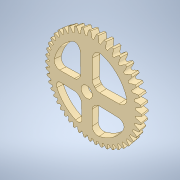
# Autodesk Inventor part: Шестерня катушки
Saved by Autodesk Inventor 2021.1 (Build 251245010, 245A)
## iProperties
Created: 2026-04-13
Part Number: Шестерня катушки
Material: Generic
Document SubType Name: Modeling
Designer: Андрей Тарасов
Density: 1 g/cm^3
Appearance: Default
Author: Андрей Тарасов
Autodesk Inventor part; units mm, degrees
(part 1 of 2)
ref_plane "YZ Plane" through (0, 0, 0) normal (1, 0, 0) x (0, 1, 0)
ref_plane "XZ Plane" through (0, 0, 0) normal (0, 1, 0) x (-1, 0, 0)
ref_plane "XY Plane" through (0, 0, 0) normal (0, 0, 1) x (1, 0, 0)
sketch "Sketch1" plane through (0, 0, 0) normal (0, 0, 1) x (1, 0, 0)
  spline S0 degree 3 poles (-2.1885, 41.8473) (-2.0953, 41.6739) (-1.9088, 41.3271) (-1.6524, 40.7949) (-1.4149, 40.2541) (-1.2364, 39.7953) (-1.1064, 39.4236) (-1.0168, 39.1423) (-0.9329, 38.8591) (-0.8777, 38.6192) (-0.8222, 38.4302) (-0.7732, 38.3167) (-0.7217, 38.2328) (-0.6774, 38.1737) (-0.6275, 38.1192) (-0.5712, 38.0711) (-0.5077, 38.0329) (-0.4402, 38.0029) (-0.3691, 37.9819) (-0.2214, 37.9693) (0, 37.9813) (0.2214, 37.9693) (0.3691, 37.9819) (0.4402, 38.0029) (0.5077, 38.0329) (0.5712, 38.0711) (0.6275, 38.1192) (0.6774, 38.1737) (0.7217, 38.2328) (0.7732, 38.3167) (0.8222, 38.4302) (0.8777, 38.6192) (0.9329, 38.8591) (1.0168, 39.1423) (1.1064, 39.4236) (1.2364, 39.7953) (1.4149, 40.2541) (1.6524, 40.7949) (1.9088, 41.3271) (2.0953, 41.6739) (2.1885, 41.8473) knots 0 0 0 0 0.059055 0.118109 0.177163 0.236216 0.265745 0.295273 0.3248 0.354329 0.36909 0.383846 0.391225 0.398597 0.405969 0.413352 0.420732 0.428104 0.435485 0.442861 0.472389 0.501917 0.509293 0.516674 0.524045 0.531426 0.538808 0.54618 0.553552 0.560931 0.575687 0.590449 0.619977 0.649505 0.679033 0.708561 0.767614 0.826668 0.885723 0.944777 0.944777 0.944777 0.944777
  circle A0 centre (0, 0) radius 37.976 construction
  circle A1 centre (0, 0) radius 37.7362 construction
  circle A2 centre (0, 0) radius 40.158 construction
  circle A3 centre (0, 0) radius 41.9045
  spline S1 degree 3 poles (-7.8664, 41.1595) (-7.7504, 41.0004) (-7.5184, 40.6823) (-7.1919, 40.19) (-6.883, 39.6865) (-6.6436, 39.2563) (-6.4643, 38.9058) (-6.3372, 38.6393) (-6.2155, 38.3701) (-6.1281, 38.14) (-6.0474, 37.9603) (-5.9835, 37.8546) (-5.921, 37.7784) (-5.8691, 37.7259) (-5.8123, 37.6787) (-5.7499, 37.6387) (-5.6818, 37.6096) (-5.6108, 37.589) (-5.5375, 37.5778) (-5.3895, 37.5855) (-5.1718, 37.6275) (-4.9508, 37.6458) (-4.8062, 37.6783) (-4.7386, 37.7089) (-4.6758, 37.7478) (-4.6181, 37.7943) (-4.5689, 37.8496) (-4.5269, 37.9104) (-4.4911, 37.975) (-4.4514, 38.0651) (-4.4184, 38.1842) (-4.3891, 38.379) (-4.3671, 38.6242) (-4.3225, 38.9162) (-4.272, 39.2071) (-4.194, 39.593) (-4.0796, 40.0719) (-3.9179, 40.64) (-3.7363, 41.2021) (-3.5988, 41.5711) (-3.5301, 41.7555) knots 0 0 0 0 0.059055 0.118109 0.177163 0.236216 0.265745 0.295273 0.3248 0.354329 0.36909 0.383846 0.391225 0.398597 0.405969 0.413352 0.420732 0.428104 0.435485 0.442861 0.472389 0.501917 0.509293 0.516674 0.524045 0.531426 0.538808 0.54618 0.553552 0.560931 0.575687 0.590449 0.619977 0.649505 0.679033 0.708561 0.767614 0.826668 0.885723 0.944777 0.944777 0.944777 0.944777
  spline S2 degree 3 poles (-13.3976, 39.705) (-13.2611, 39.5632) (-12.988, 39.2796) (-12.5975, 38.8363) (-12.2229, 38.3797) (-11.9272, 37.9861) (-11.7018, 37.6632) (-11.5396, 37.4165) (-11.3823, 37.1664) (-11.2645, 36.9503) (-11.16, 36.7833) (-11.0823, 36.6872) (-11.01, 36.6203) (-10.9514, 36.5753) (-10.8887, 36.5363) (-10.8215, 36.5052) (-10.75, 36.4856) (-10.6769, 36.4749) (-10.6027, 36.4738) (-10.4572, 36.5016) (-10.2472, 36.5728) (-10.0308, 36.6211) (-9.892, 36.673) (-9.8292, 36.7124) (-9.7723, 36.7596) (-9.7214, 36.8134) (-9.6802, 36.8749) (-9.6468, 36.9409) (-9.6202, 37.0097) (-9.5932, 37.1045) (-9.5767, 37.227) (-9.5742, 37.4239) (-9.5858, 37.6698) (-9.5814, 37.9651) (-9.571, 38.2602) (-9.5461, 38.6532) (-9.498, 39.1431) (-9.4152, 39.728) (-9.3119, 40.3096) (-9.2259, 40.6938) (-9.1829, 40.8859) knots 0 0 0 0 0.059055 0.118109 0.177163 0.236216 0.265745 0.295273 0.3248 0.354329 0.36909 0.383846 0.391225 0.398597 0.405969 0.413352 0.420732 0.428104 0.435485 0.442861 0.472389 0.501917 0.509293 0.516674 0.524045 0.531426 0.538808 0.54618 0.553552 0.560931 0.575687 0.590449 0.619977 0.649505 0.679033 0.708561 0.767614 0.826668 0.885723 0.944777 0.944777 0.944777 0.944777
  spline S3 degree 3 poles (-18.6793, 37.5109) (-18.5248, 37.389) (-18.2156, 37.1452) (-17.7683, 36.7593) (-17.335, 36.3579) (-16.9885, 36.0082) (-16.7213, 35.719) (-16.527, 35.4967) (-16.3371, 35.2703) (-16.1909, 35.0723) (-16.0647, 34.9211) (-15.9747, 34.8365) (-15.8939, 34.7801) (-15.8298, 34.7434) (-15.7623, 34.7133) (-15.6915, 34.6916) (-15.618, 34.682) (-15.5442, 34.6813) (-15.4705, 34.6904) (-15.3301, 34.7377) (-15.1318, 34.8369) (-14.9239, 34.9141) (-14.7935, 34.9844) (-14.7366, 35.0321) (-14.6867, 35.0865) (-14.6436, 35.1468) (-14.6111, 35.2134) (-14.5871, 35.2832) (-14.5701, 35.3551) (-14.5562, 35.4526) (-14.5566, 35.5762) (-14.5809, 35.7716) (-14.6259, 36.0136) (-14.6617, 36.3069) (-14.6916, 36.6006) (-14.7205, 36.9933) (-14.7395, 37.4852) (-14.7372, 38.0759) (-14.714, 38.6662) (-14.6811, 39.0585) (-14.6647, 39.2547) knots 0 0 0 0 0.059055 0.118109 0.177163 0.236216 0.265745 0.295273 0.3248 0.354329 0.36909 0.383846 0.391225 0.398597 0.405969 0.413352 0.420732 0.428104 0.435485 0.442861 0.472389 0.501917 0.509293 0.516674 0.524045 0.531426 0.538808 0.54618 0.553552 0.560931 0.575687 0.590449 0.619977 0.649505 0.679033 0.708561 0.767614 0.826668 0.885723 0.944777 0.944777 0.944777 0.944777
  spline S4 degree 3 poles (-23.6131, 34.618) (-23.4433, 34.5183) (-23.1038, 34.3189) (-22.6082, 33.9974) (-22.1243, 33.6588) (-21.7334, 33.3595) (-21.4293, 33.1094) (-21.2065, 32.9156) (-20.9876, 32.7173) (-20.8158, 32.541) (-20.6702, 32.4084) (-20.5694, 32.3368) (-20.4818, 32.2919) (-20.4132, 32.2643) (-20.3423, 32.2437) (-20.2692, 32.2319) (-20.1951, 32.2323) (-20.1218, 32.2417) (-20.0501, 32.2607) (-19.9175, 32.3267) (-19.7345, 32.452) (-19.539, 32.5568) (-19.4194, 32.6442) (-19.3696, 32.6991) (-19.3275, 32.7599) (-19.2931, 32.8255) (-19.2699, 32.8958) (-19.2556, 32.9683) (-19.2486, 33.0418) (-19.2481, 33.1403) (-19.2653, 33.2627) (-19.316, 33.453) (-19.3935, 33.6866) (-19.4689, 33.9723) (-19.5385, 34.2592) (-19.6207, 34.6443) (-19.7065, 35.1291) (-19.7846, 35.7145) (-19.842, 36.3025) (-19.8628, 36.6957) (-19.8733, 36.8923) knots 0 0 0 0 0.059055 0.118109 0.177163 0.236216 0.265745 0.295273 0.3248 0.354329 0.36909 0.383846 0.391225 0.398597 0.405969 0.413352 0.420732 0.428104 0.435485 0.442861 0.472389 0.501917 0.509293 0.516674 0.524045 0.531426 0.538808 0.54618 0.553552 0.560931 0.575687 0.590449 0.619977 0.649505 0.679033 0.708561 0.767614 0.826668 0.885723 0.944777 0.944777 0.944777 0.944777
  spline S5 degree 3 poles (-28.107, 31.0803) (-27.9252, 31.0046) (-27.5617, 30.8533) (-27.027, 30.6023) (-26.5014, 30.3327) (-26.0734, 30.0894) (-25.7381, 29.8831) (-25.491, 29.7214) (-25.2471, 29.5547) (-25.0529, 29.4035) (-24.8906, 29.2919) (-24.781, 29.2347) (-24.6881, 29.2022) (-24.6164, 29.1842) (-24.5433, 29.1734) (-24.4693, 29.1717) (-24.396, 29.1822) (-24.3246, 29.2015) (-24.2562, 29.23) (-24.1338, 29.3135) (-23.9695, 29.4625) (-23.7902, 29.593) (-23.6836, 29.6959) (-23.6417, 29.7571) (-23.6083, 29.823) (-23.5831, 29.8926) (-23.5698, 29.9655) (-23.5655, 30.0393) (-23.5685, 30.1131) (-23.5814, 30.2107) (-23.6151, 30.3296) (-23.6913, 30.5112) (-23.7999, 30.7321) (-23.9135, 31.0048) (-24.0215, 31.2796) (-24.1553, 31.6499) (-24.3064, 32.1185) (-24.4634, 32.6879) (-24.6004, 33.2625) (-24.6746, 33.6492) (-24.7117, 33.8426) knots 0 0 0 0 0.059055 0.118109 0.177163 0.236216 0.265745 0.295273 0.3248 0.354329 0.36909 0.383846 0.391225 0.398597 0.405969 0.413352 0.420732 0.428104 0.435485 0.442861 0.472389 0.501917 0.509293 0.516674 0.524045 0.531426 0.538808 0.54618 0.553552 0.560931 0.575687 0.590449 0.619977 0.649505 0.679033 0.708561 0.767614 0.826668 0.885723 0.944777 0.944777 0.944777 0.944777
  spline S6 degree 3 poles (-32.0773, 26.9635) (-31.8869, 26.9133) (-31.5062, 26.8129) (-30.9423, 26.6371) (-30.3849, 26.4415) (-29.9277, 26.2589) (-29.5674, 26.1001) (-29.3006, 25.9736) (-29.0363, 25.8416) (-28.8234, 25.7182) (-28.6474, 25.6298) (-28.531, 25.5881) (-28.4345, 25.5685) (-28.3611, 25.5605) (-28.2872, 25.5597) (-28.2136, 25.5681) (-28.1424, 25.5885) (-28.0744, 25.6173) (-28.0104, 25.6549) (-27.9005, 25.7542) (-27.7581, 25.9243) (-27.5982, 26.0779) (-27.5066, 26.1943) (-27.4734, 26.2607) (-27.4493, 26.3306) (-27.4338, 26.403) (-27.4305, 26.477) (-27.4363, 26.5506) (-27.4493, 26.6233) (-27.4755, 26.7183) (-27.525, 26.8315) (-27.6252, 27.0011) (-27.7629, 27.2052) (-27.9126, 27.4598) (-28.057, 27.7174) (-28.24, 28.066) (-28.4534, 28.5096) (-28.6866, 29.0523) (-28.9005, 29.603) (-29.0266, 29.976) (-29.0897, 30.1625) knots 0 0 0 0 0.059055 0.118109 0.177163 0.236216 0.265745 0.295273 0.3248 0.354329 0.36909 0.383846 0.391225 0.398597 0.405969 0.413352 0.420732 0.428104 0.435485 0.442861 0.472389 0.501917 0.509293 0.516674 0.524045 0.531426 0.538808 0.54618 0.553552 0.560931 0.575687 0.590449 0.619977 0.649505 0.679033 0.708561 0.767614 0.826668 0.885723 0.944777 0.944777 0.944777 0.944777
  spline S7 degree 3 poles (-35.4501, 22.3445) (-35.2546, 22.3207) (-34.8638, 22.2731) (-34.2811, 22.1757) (-33.7024, 22.0578) (-33.2246, 21.9391) (-32.846, 21.8309) (-32.5645, 21.7419) (-32.2847, 21.6472) (-32.0569, 21.5539) (-31.8705, 21.4903) (-31.7495, 21.4648) (-31.6512, 21.4585) (-31.5774, 21.4606) (-31.5041, 21.4699) (-31.4323, 21.4882) (-31.3646, 21.5181) (-31.3011, 21.5559) (-31.2429, 21.6019) (-31.1475, 21.7153) (-31.0296, 21.9031) (-30.8921, 22.0771) (-30.8172, 22.2049) (-30.7934, 22.2752) (-30.779, 22.3476) (-30.7735, 22.4215) (-30.7803, 22.4953) (-30.7961, 22.5674) (-30.8189, 22.6377) (-30.8577, 22.7282) (-30.9222, 22.8336) (-31.0446, 22.988) (-31.2087, 23.1714) (-31.3917, 23.4033) (-31.5699, 23.6388) (-31.7986, 23.9593) (-32.0705, 24.3697) (-32.3753, 24.8756) (-32.6622, 25.392) (-32.838, 25.7443) (-32.9259, 25.9205) knots 0 0 0 0 0.059055 0.118109 0.177163 0.236216 0.265745 0.295273 0.3248 0.354329 0.36909 0.383846 0.391225 0.398597 0.405969 0.413352 0.420732 0.428104 0.435485 0.442861 0.472389 0.501917 0.509293 0.516674 0.524045 0.531426 0.538808 0.54618 0.553552 0.560931 0.575687 0.590449 0.619977 0.649505 0.679033 0.708561 0.767614 0.826668 0.885723 0.944777 0.944777 0.944777 0.944777
  spline S8 degree 3 poles (-38.1625, 17.3093) (-37.9656, 17.3123) (-37.5719, 17.3184) (-36.9814, 17.3012) (-36.392, 17.2633) (-35.9025, 17.2107) (-35.5127, 17.155) (-35.2217, 17.1052) (-34.9316, 17.0494) (-34.6932, 16.9881) (-34.4999, 16.9504) (-34.3766, 16.9416) (-34.2784, 16.9488) (-34.2055, 16.9609) (-34.1342, 16.9801) (-34.0655, 17.008) (-34.0025, 17.0468) (-33.9447, 17.093) (-33.8933, 17.1464) (-33.8143, 17.2717) (-33.723, 17.4739) (-33.6105, 17.665) (-33.5537, 17.8018) (-33.5397, 17.8747) (-33.5353, 17.9484) (-33.5399, 18.0223) (-33.5567, 18.0945) (-33.5822, 18.1639) (-33.6143, 18.2303) (-33.6651, 18.3147) (-33.7434, 18.4104) (-33.8856, 18.5466) (-34.0732, 18.706) (-34.2861, 18.9108) (-34.4946, 19.1198) (-34.7649, 19.4062) (-35.0901, 19.7758) (-35.461, 20.2355) (-35.8156, 20.708) (-36.0377, 21.0331) (-36.1487, 21.1956) knots 0 0 0 0 0.059055 0.118109 0.177163 0.236216 0.265745 0.295273 0.3248 0.354329 0.36909 0.383846 0.391225 0.398597 0.405969 0.413352 0.420732 0.428104 0.435485 0.442861 0.472389 0.501917 0.509293 0.516674 0.524045 0.531426 0.538808 0.54618 0.553552 0.560931 0.575687 0.590449 0.619977 0.649505 0.679033 0.708561 0.767614 0.826668 0.885723 0.944777 0.944777 0.944777 0.944777
  spline S9 degree 3 poles (-40.164, 11.9516) (-39.9694, 11.9814) (-39.5802, 12.041) (-38.9928, 12.1044) (-38.4037, 12.1471) (-37.9116, 12.1617) (-37.5179, 12.1596) (-37.2228, 12.1499) (-36.9278, 12.1341) (-36.6833, 12.1058) (-36.4866, 12.0948) (-36.3633, 12.1029) (-36.267, 12.1234) (-36.1964, 12.1453) (-36.1284, 12.174) (-36.0642, 12.211) (-36.007, 12.2581) (-35.9561, 12.3116) (-35.9124, 12.3716) (-35.8512, 12.5065) (-35.7883, 12.7192) (-35.7029, 12.9238) (-35.6652, 13.0671) (-35.6612, 13.1412) (-35.6669, 13.2149) (-35.6816, 13.2875) (-35.7081, 13.3566) (-35.7427, 13.4219) (-35.7836, 13.4834) (-35.8454, 13.5601) (-35.936, 13.6442) (-36.0954, 13.7598) (-36.303, 13.8921) (-36.5417, 14.0661) (-36.7768, 14.2447) (-37.0836, 14.4916) (-37.4561, 14.8135) (-37.8861, 15.2184) (-38.3017, 15.6382) (-38.566, 15.9301) (-38.6982, 16.076) knots 0 0 0 0 0.059055 0.118109 0.177163 0.236216 0.265745 0.295273 0.3248 0.354329 0.36909 0.383846 0.391225 0.398597 0.405969 0.413352 0.420732 0.428104 0.435485 0.442861 0.472389 0.501917 0.509293 0.516674 0.524045 0.531426 0.538808 0.54618 0.553552 0.560931 0.575687 0.590449 0.619977 0.649505 0.679033 0.708561 0.767614 0.826668 0.885723 0.944777 0.944777 0.944777 0.944777
  spline S10 degree 3 poles (-41.4173, 6.3713) (-41.2286, 6.4273) (-40.8511, 6.5394) (-40.2779, 6.6821) (-39.7, 6.8046) (-39.2145, 6.8861) (-38.8242, 6.9377) (-38.5305, 6.9682) (-38.2361, 6.9928) (-37.99, 6.998) (-37.7937, 7.0139) (-37.6726, 7.0387) (-37.58, 7.0721) (-37.5131, 7.1034) (-37.4496, 7.1412) (-37.391, 7.1865) (-37.3407, 7.2409) (-37.2976, 7.3009) (-37.2625, 7.3663) (-37.2202, 7.5083) (-37.1869, 7.7275) (-37.1301, 7.9419) (-37.1123, 8.089) (-37.1185, 8.1629) (-37.1342, 8.2351) (-37.1586, 8.3051) (-37.1942, 8.37) (-37.2374, 8.4299) (-37.2863, 8.4853) (-37.358, 8.5528) (-37.4592, 8.6238) (-37.6329, 8.7166) (-37.8565, 8.8195) (-38.1167, 8.9593) (-38.374, 9.1043) (-38.7114, 9.3071) (-39.1243, 9.5752) (-39.6055, 9.9178) (-40.0744, 10.2771) (-40.376, 10.5303) (-40.5267, 10.6568) knots 0 0 0 0 0.059055 0.118109 0.177163 0.236216 0.265745 0.295273 0.3248 0.354329 0.36909 0.383846 0.391225 0.398597 0.405969 0.413352 0.420732 0.428104 0.435485 0.442861 0.472389 0.501917 0.509293 0.516674 0.524045 0.531426 0.538808 0.54618 0.553552 0.560931 0.575687 0.590449 0.619977 0.649505 0.679033 0.708561 0.767614 0.826668 0.885723 0.944777 0.944777 0.944777 0.944777
  spline S11 degree 3 poles (-41.8991, 0.6723) (-41.7197, 0.7535) (-41.361, 0.9159) (-40.8126, 1.1354) (-40.2568, 1.3354) (-39.7869, 1.4823) (-39.4072, 1.5865) (-39.1204, 1.6567) (-38.8322, 1.7212) (-38.5891, 1.7598) (-38.3968, 1.8023) (-38.2802, 1.8434) (-38.1929, 1.8891) (-38.1309, 1.9292) (-38.0731, 1.9753) (-38.0213, 2.0282) (-37.9789, 2.0889) (-37.9444, 2.1542) (-37.9185, 2.2238) (-37.8959, 2.3702) (-37.8927, 2.5919) (-37.8657, 2.812) (-37.8681, 2.9602) (-37.8843, 3.0326) (-37.9096, 3.102) (-37.9433, 3.1679) (-37.9875, 3.2274) (-38.0385, 3.2809) (-38.0944, 3.3291) (-38.1746, 3.3863) (-38.2845, 3.4428) (-38.4693, 3.5111) (-38.7048, 3.5825) (-38.9817, 3.6856) (-39.2562, 3.7942) (-39.6182, 3.9492) (-40.0637, 4.1586) (-40.5871, 4.4325) (-41.1005, 4.7246) (-41.4338, 4.9343) (-41.6004, 5.0392) knots 0 0 0 0 0.059055 0.118109 0.177163 0.236216 0.265745 0.295273 0.3248 0.354329 0.36909 0.383846 0.391225 0.398597 0.405969 0.413352 0.420732 0.428104 0.435485 0.442861 0.472389 0.501917 0.509293 0.516674 0.524045 0.531426 0.538808 0.54618 0.553552 0.560931 0.575687 0.590449 0.619977 0.649505 0.679033 0.708561 0.767614 0.826668 0.885723 0.944777 0.944777 0.944777 0.944777
  spline S12 degree 3 poles (-41.6004, -5.0392) (-41.4338, -4.9343) (-41.1005, -4.7246) (-40.5871, -4.4325) (-40.0637, -4.1586) (-39.6182, -3.9492) (-39.2562, -3.7942) (-38.9817, -3.6856) (-38.7048, -3.5825) (-38.4693, -3.5111) (-38.2845, -3.4428) (-38.1746, -3.3863) (-38.0944, -3.3291) (-38.0385, -3.2809) (-37.9875, -3.2274) (-37.9433, -3.1679) (-37.9096, -3.102) (-37.8843, -3.0326) (-37.8681, -2.9602) (-37.8657, -2.812) (-37.8927, -2.5919) (-37.8959, -2.3702) (-37.9185, -2.2238) (-37.9444, -2.1542) (-37.9789, -2.0889) (-38.0213, -2.0282) (-38.0731, -1.9753) (-38.1309, -1.9292) (-38.1929, -1.8891) (-38.2802, -1.8434) (-38.3968, -1.8023) (-38.5891, -1.7598) (-38.8322, -1.7212) (-39.1204, -1.6567) (-39.4072, -1.5865) (-39.7869, -1.4823) (-40.2568, -1.3354) (-40.8126, -1.1354) (-41.361, -0.9159) (-41.7197, -0.7535) (-41.8991, -0.6723) knots 0 0 0 0 0.059055 0.118109 0.177163 0.236216 0.265745 0.295273 0.3248 0.354329 0.36909 0.383846 0.391225 0.398597 0.405969 0.413352 0.420732 0.428104 0.435485 0.442861 0.472389 0.501917 0.509293 0.516674 0.524045 0.531426 0.538808 0.54618 0.553552 0.560931 0.575687 0.590449 0.619977 0.649505 0.679033 0.708561 0.767614 0.826668 0.885723 0.944777 0.944777 0.944777 0.944777
  spline S13 degree 3 poles (-40.5267, -10.6568) (-40.376, -10.5303) (-40.0744, -10.2771) (-39.6055, -9.9178) (-39.1243, -9.5752) (-38.7114, -9.3071) (-38.374, -9.1043) (-38.1167, -8.9593) (-37.8565, -8.8195) (-37.6329, -8.7166) (-37.4592, -8.6238) (-37.358, -8.5528) (-37.2863, -8.4853) (-37.2374, -8.4299) (-37.1942, -8.37) (-37.1586, -8.3051) (-37.1342, -8.2351) (-37.1185, -8.1629) (-37.1123, -8.089) (-37.1301, -7.9419) (-37.1869, -7.7275) (-37.2202, -7.5083) (-37.2625, -7.3663) (-37.2976, -7.3009) (-37.3407, -7.2409) (-37.391, -7.1865) (-37.4496, -7.1412) (-37.5131, -7.1034) (-37.58, -7.0721) (-37.6726, -7.0387) (-37.7937, -7.0139) (-37.99, -6.998) (-38.2361, -6.9928) (-38.5305, -6.9682) (-38.8242, -6.9377) (-39.2145, -6.8861) (-39.7, -6.8046) (-40.2779, -6.6821) (-40.8511, -6.5394) (-41.2286, -6.4273) (-41.4173, -6.3713) knots 0 0 0 0 0.059055 0.118109 0.177163 0.236216 0.265745 0.295273 0.3248 0.354329 0.36909 0.383846 0.391225 0.398597 0.405969 0.413352 0.420732 0.428104 0.435485 0.442861 0.472389 0.501917 0.509293 0.516674 0.524045 0.531426 0.538808 0.54618 0.553552 0.560931 0.575687 0.590449 0.619977 0.649505 0.679033 0.708561 0.767614 0.826668 0.885723 0.944777 0.944777 0.944777 0.944777
  spline S14 degree 3 poles (-38.6982, -16.076) (-38.566, -15.9301) (-38.3017, -15.6382) (-37.8861, -15.2184) (-37.4561, -14.8135) (-37.0836, -14.4916) (-36.7768, -14.2447) (-36.5417, -14.0661) (-36.303, -13.8921) (-36.0954, -13.7598) (-35.936, -13.6442) (-35.8454, -13.5601) (-35.7836, -13.4834) (-35.7427, -13.4219) (-35.7081, -13.3566) (-35.6816, -13.2875) (-35.6669, -13.2149) (-35.6612, -13.1412) (-35.6652, -13.0671) (-35.7029, -12.9238) (-35.7883, -12.7192) (-35.8512, -12.5065) (-35.9124, -12.3716) (-35.9561, -12.3116) (-36.007, -12.2581) (-36.0642, -12.211) (-36.1284, -12.174) (-36.1964, -12.1453) (-36.267, -12.1234) (-36.3633, -12.1029) (-36.4866, -12.0948) (-36.6833, -12.1058) (-36.9278, -12.1341) (-37.2228, -12.1499) (-37.5179, -12.1596) (-37.9116, -12.1617) (-38.4037, -12.1471) (-38.9928, -12.1044) (-39.5802, -12.041) (-39.9694, -11.9814) (-40.164, -11.9516) knots 0 0 0 0 0.059055 0.118109 0.177163 0.236216 0.265745 0.295273 0.3248 0.354329 0.36909 0.383846 0.391225 0.398597 0.405969 0.413352 0.420732 0.428104 0.435485 0.442861 0.472389 0.501917 0.509293 0.516674 0.524045 0.531426 0.538808 0.54618 0.553552 0.560931 0.575687 0.590449 0.619977 0.649505 0.679033 0.708561 0.767614 0.826668 0.885723 0.944777 0.944777 0.944777 0.944777
  spline S15 degree 3 poles (-36.1487, -21.1956) (-36.0377, -21.0331) (-35.8156, -20.708) (-35.461, -20.2355) (-35.0901, -19.7758) (-34.7649, -19.4062) (-34.4946, -19.1198) (-34.2861, -18.9108) (-34.0732, -18.706) (-33.8856, -18.5466) (-33.7434, -18.4104) (-33.6651, -18.3147) (-33.6143, -18.2303) (-33.5822, -18.1639) (-33.5567, -18.0945) (-33.5399, -18.0223) (-33.5353, -17.9484) (-33.5397, -17.8747) (-33.5537, -17.8018) (-33.6105, -17.665) (-33.723, -17.4739) (-33.8143, -17.2717) (-33.8933, -17.1464) (-33.9447, -17.093) (-34.0025, -17.0468) (-34.0655, -17.008) (-34.1342, -16.9801) (-34.2055, -16.9609) (-34.2784, -16.9488) (-34.3766, -16.9416) (-34.4999, -16.9504) (-34.6932, -16.9881) (-34.9316, -17.0494) (-35.2217, -17.1052) (-35.5127, -17.155) (-35.9025, -17.2107) (-36.392, -17.2633) (-36.9814, -17.3012) (-37.5719, -17.3184) (-37.9656, -17.3123) (-38.1625, -17.3093) knots 0 0 0 0 0.059055 0.118109 0.177163 0.236216 0.265745 0.295273 0.3248 0.354329 0.36909 0.383846 0.391225 0.398597 0.405969 0.413352 0.420732 0.428104 0.435485 0.442861 0.472389 0.501917 0.509293 0.516674 0.524045 0.531426 0.538808 0.54618 0.553552 0.560931 0.575687 0.590449 0.619977 0.649505 0.679033 0.708561 0.767614 0.826668 0.885723 0.944777 0.944777 0.944777 0.944777
  spline S16 degree 3 poles (-32.9259, -25.9205) (-32.838, -25.7443) (-32.6622, -25.392) (-32.3753, -24.8756) (-32.0705, -24.3697) (-31.7986, -23.9593) (-31.5699, -23.6388) (-31.3917, -23.4033) (-31.2087, -23.1714) (-31.0446, -22.988) (-30.9222, -22.8336) (-30.8577, -22.7282) (-30.8189, -22.6377) (-30.7961, -22.5674) (-30.7803, -22.4953) (-30.7735, -22.4215) (-30.779, -22.3476) (-30.7934, -22.2752) (-30.8172, -22.2049) (-30.8921, -22.0771) (-31.0296, -21.9031) (-31.1475, -21.7153) (-31.2429, -21.6019) (-31.3011, -21.5559) (-31.3646, -21.5181) (-31.4323, -21.4882) (-31.5041, -21.4699) (-31.5774, -21.4606) (-31.6512, -21.4585) (-31.7495, -21.4648) (-31.8705, -21.4903) (-32.0569, -21.5539) (-32.2847, -21.6472) (-32.5645, -21.7419) (-32.846, -21.8309) (-33.2246, -21.9391) (-33.7024, -22.0578) (-34.2811, -22.1757) (-34.8638, -22.2731) (-35.2546, -22.3207) (-35.4501, -22.3445) knots 0 0 0 0 0.059055 0.118109 0.177163 0.236216 0.265745 0.295273 0.3248 0.354329 0.36909 0.383846 0.391225 0.398597 0.405969 0.413352 0.420732 0.428104 0.435485 0.442861 0.472389 0.501917 0.509293 0.516674 0.524045 0.531426 0.538808 0.54618 0.553552 0.560931 0.575687 0.590449 0.619977 0.649505 0.679033 0.708561 0.767614 0.826668 0.885723 0.944777 0.944777 0.944777 0.944777
  spline S17 degree 3 poles (-29.0897, -30.1625) (-29.0266, -29.976) (-28.9005, -29.603) (-28.6866, -29.0523) (-28.4534, -28.5096) (-28.24, -28.066) (-28.057, -27.7174) (-27.9126, -27.4598) (-27.7629, -27.2052) (-27.6252, -27.0011) (-27.525, -26.8315) (-27.4755, -26.7183) (-27.4493, -26.6233) (-27.4363, -26.5506) (-27.4305, -26.477) (-27.4338, -26.403) (-27.4493, -26.3306) (-27.4734, -26.2607) (-27.5066, -26.1943) (-27.5982, -26.0779) (-27.7581, -25.9243) (-27.9005, -25.7542) (-28.0104, -25.6549) (-28.0744, -25.6173) (-28.1424, -25.5885) (-28.2136, -25.5681) (-28.2872, -25.5597) (-28.3611, -25.5605) (-28.4345, -25.5685) (-28.531, -25.5881) (-28.6474, -25.6298) (-28.8234, -25.7182) (-29.0363, -25.8416) (-29.3006, -25.9736) (-29.5674, -26.1001) (-29.9277, -26.2589) (-30.3849, -26.4415) (-30.9423, -26.6371) (-31.5062, -26.8129) (-31.8869, -26.9133) (-32.0773, -26.9635) knots 0 0 0 0 0.059055 0.118109 0.177163 0.236216 0.265745 0.295273 0.3248 0.354329 0.36909 0.383846 0.391225 0.398597 0.405969 0.413352 0.420732 0.428104 0.435485 0.442861 0.472389 0.501917 0.509293 0.516674 0.524045 0.531426 0.538808 0.54618 0.553552 0.560931 0.575687 0.590449 0.619977 0.649505 0.679033 0.708561 0.767614 0.826668 0.885723 0.944777 0.944777 0.944777 0.944777
  spline S18 degree 3 poles (-24.7117, -33.8426) (-24.6746, -33.6492) (-24.6004, -33.2625) (-24.4634, -32.6879) (-24.3064, -32.1185) (-24.1553, -31.6499) (-24.0215, -31.2796) (-23.9135, -31.0048) (-23.7999, -30.7321) (-23.6913, -30.5112) (-23.6151, -30.3296) (-23.5814, -30.2107) (-23.5685, -30.1131) (-23.5655, -30.0393) (-23.5698, -29.9655) (-23.5831, -29.8926) (-23.6083, -29.823) (-23.6417, -29.7571) (-23.6836, -29.6959) (-23.7902, -29.593) (-23.9695, -29.4625) (-24.1338, -29.3135) (-24.2562, -29.23) (-24.3246, -29.2015) (-24.396, -29.1822) (-24.4693, -29.1717) (-24.5433, -29.1734) (-24.6164, -29.1842) (-24.6881, -29.2022) (-24.781, -29.2347) (-24.8906, -29.2919) (-25.0529, -29.4035) (-25.2471, -29.5547) (-25.491, -29.7214) (-25.7381, -29.8831) (-26.0734, -30.0894) (-26.5014, -30.3327) (-27.027, -30.6023) (-27.5617, -30.8533) (-27.9252, -31.0046) (-28.107, -31.0803) knots 0 0 0 0 0.059055 0.118109 0.177163 0.236216 0.265745 0.295273 0.3248 0.354329 0.36909 0.383846 0.391225 0.398597 0.405969 0.413352 0.420732 0.428104 0.435485 0.442861 0.472389 0.501917 0.509293 0.516674 0.524045 0.531426 0.538808 0.54618 0.553552 0.560931 0.575687 0.590449 0.619977 0.649505 0.679033 0.708561 0.767614 0.826668 0.885723 0.944777 0.944777 0.944777 0.944777
  spline S19 degree 3 poles (-19.8733, -36.8923) (-19.8628, -36.6957) (-19.842, -36.3025) (-19.7846, -35.7145) (-19.7065, -35.1291) (-19.6207, -34.6443) (-19.5385, -34.2592) (-19.4689, -33.9723) (-19.3935, -33.6866) (-19.316, -33.453) (-19.2653, -33.2627) (-19.2481, -33.1403) (-19.2486, -33.0418) (-19.2556, -32.9683) (-19.2699, -32.8958) (-19.2931, -32.8255) (-19.3275, -32.7599) (-19.3696, -32.6991) (-19.4194, -32.6442) (-19.539, -32.5568) (-19.7345, -32.452) (-19.9175, -32.3267) (-20.0501, -32.2607) (-20.1218, -32.2417) (-20.1951, -32.2323) (-20.2692, -32.2319) (-20.3423, -32.2437) (-20.4132, -32.2643) (-20.4818, -32.2919) (-20.5694, -32.3368) (-20.6702, -32.4084) (-20.8158, -32.541) (-20.9876, -32.7173) (-21.2065, -32.9156) (-21.4293, -33.1094) (-21.7334, -33.3595) (-22.1243, -33.6588) (-22.6082, -33.9974) (-23.1038, -34.3189) (-23.4433, -34.5183) (-23.6131, -34.618) knots 0 0 0 0 0.059055 0.118109 0.177163 0.236216 0.265745 0.295273 0.3248 0.354329 0.36909 0.383846 0.391225 0.398597 0.405969 0.413352 0.420732 0.428104 0.435485 0.442861 0.472389 0.501917 0.509293 0.516674 0.524045 0.531426 0.538808 0.54618 0.553552 0.560931 0.575687 0.590449 0.619977 0.649505 0.679033 0.708561 0.767614 0.826668 0.885723 0.944777 0.944777 0.944777 0.944777
  spline S20 degree 3 poles (-14.6647, -39.2547) (-14.6811, -39.0585) (-14.714, -38.6662) (-14.7372, -38.0759) (-14.7395, -37.4852) (-14.7205, -36.9933) (-14.6916, -36.6006) (-14.6617, -36.3069) (-14.6259, -36.0136) (-14.5809, -35.7716) (-14.5566, -35.5762) (-14.5562, -35.4526) (-14.5701, -35.3551) (-14.5871, -35.2832) (-14.6111, -35.2134) (-14.6436, -35.1468) (-14.6867, -35.0865) (-14.7366, -35.0321) (-14.7935, -34.9844) (-14.9239, -34.9141) (-15.1318, -34.8369) (-15.3301, -34.7377) (-15.4705, -34.6904) (-15.5442, -34.6813) (-15.618, -34.682) (-15.6915, -34.6916) (-15.7623, -34.7133) (-15.8298, -34.7434) (-15.8939, -34.7801) (-15.9747, -34.8365) (-16.0647, -34.9211) (-16.1909, -35.0723) (-16.3371, -35.2703) (-16.527, -35.4967) (-16.7213, -35.719) (-16.9885, -36.0082) (-17.335, -36.3579) (-17.7683, -36.7593) (-18.2156, -37.1452) (-18.5248, -37.389) (-18.6793, -37.5109) knots 0 0 0 0 0.059055 0.118109 0.177163 0.236216 0.265745 0.295273 0.3248 0.354329 0.36909 0.383846 0.391225 0.398597 0.405969 0.413352 0.420732 0.428104 0.435485 0.442861 0.472389 0.501917 0.509293 0.516674 0.524045 0.531426 0.538808 0.54618 0.553552 0.560931 0.575687 0.590449 0.619977 0.649505 0.679033 0.708561 0.767614 0.826668 0.885723 0.944777 0.944777 0.944777 0.944777
  spline S21 degree 3 poles (-9.1829, -40.8859) (-9.2259, -40.6938) (-9.3119, -40.3096) (-9.4152, -39.728) (-9.498, -39.1431) (-9.5461, -38.6532) (-9.571, -38.2602) (-9.5814, -37.9651) (-9.5858, -37.6698) (-9.5742, -37.4239) (-9.5767, -37.227) (-9.5932, -37.1045) (-9.6202, -37.0097) (-9.6468, -36.9409) (-9.6802, -36.8749) (-9.7214, -36.8134) (-9.7723, -36.7596) (-9.8292, -36.7124) (-9.892, -36.673) (-10.0308, -36.6211) (-10.2472, -36.5728) (-10.4572, -36.5016) (-10.6027, -36.4738) (-10.6769, -36.4749) (-10.75, -36.4856) (-10.8215, -36.5052) (-10.8887, -36.5363) (-10.9514, -36.5753) (-11.01, -36.6203) (-11.0823, -36.6872) (-11.16, -36.7833) (-11.2645, -36.9503) (-11.3823, -37.1664) (-11.5396, -37.4165) (-11.7018, -37.6632) (-11.9272, -37.9861) (-12.2229, -38.3797) (-12.5975, -38.8363) (-12.988, -39.2796) (-13.2611, -39.5632) (-13.3976, -39.705) knots 0 0 0 0 0.059055 0.118109 0.177163 0.236216 0.265745 0.295273 0.3248 0.354329 0.36909 0.383846 0.391225 0.398597 0.405969 0.413352 0.420732 0.428104 0.435485 0.442861 0.472389 0.501917 0.509293 0.516674 0.524045 0.531426 0.538808 0.54618 0.553552 0.560931 0.575687 0.590449 0.619977 0.649505 0.679033 0.708561 0.767614 0.826668 0.885723 0.944777 0.944777 0.944777 0.944777
  spline S22 degree 3 poles (-3.5301, -41.7555) (-3.5988, -41.5711) (-3.7363, -41.2021) (-3.9179, -40.64) (-4.0796, -40.0719) (-4.194, -39.593) (-4.272, -39.2071) (-4.3225, -38.9162) (-4.3671, -38.6242) (-4.3891, -38.379) (-4.4184, -38.1842) (-4.4514, -38.0651) (-4.4911, -37.975) (-4.5269, -37.9104) (-4.5689, -37.8496) (-4.6181, -37.7943) (-4.6758, -37.7478) (-4.7386, -37.7089) (-4.8062, -37.6783) (-4.9508, -37.6458) (-5.1718, -37.6275) (-5.3895, -37.5855) (-5.5375, -37.5778) (-5.6108, -37.589) (-5.6818, -37.6096) (-5.7499, -37.6387) (-5.8123, -37.6787) (-5.8691, -37.7259) (-5.921, -37.7784) (-5.9835, -37.8546) (-6.0474, -37.9603) (-6.1281, -38.14) (-6.2155, -38.3701) (-6.3372, -38.6393) (-6.4643, -38.9058) (-6.6436, -39.2563) (-6.883, -39.6865) (-7.1919, -40.19) (-7.5184, -40.6823) (-7.7504, -41.0004) (-7.8664, -41.1595) knots 0 0 0 0 0.059055 0.118109 0.177163 0.236216 0.265745 0.295273 0.3248 0.354329 0.36909 0.383846 0.391225 0.398597 0.405969 0.413352 0.420732 0.428104 0.435485 0.442861 0.472389 0.501917 0.509293 0.516674 0.524045 0.531426 0.538808 0.54618 0.553552 0.560931 0.575687 0.590449 0.619977 0.649505 0.679033 0.708561 0.767614 0.826668 0.885723 0.944777 0.944777 0.944777 0.944777
  spline S23 degree 3 poles (2.1885, -41.8473) (2.0953, -41.6739) (1.9088, -41.3271) (1.6524, -40.7949) (1.4149, -40.2541) (1.2364, -39.7953) (1.1064, -39.4236) (1.0168, -39.1423) (0.9329, -38.8591) (0.8777, -38.6192) (0.8222, -38.4302) (0.7732, -38.3167) (0.7217, -38.2328) (0.6774, -38.1737) (0.6275, -38.1192) (0.5712, -38.0711) (0.5077, -38.0329) (0.4402, -38.0029) (0.3691, -37.9819) (0.2214, -37.9693) (0, -37.9813) (-0.2214, -37.9693) (-0.3691, -37.9819) (-0.4402, -38.0029) (-0.5077, -38.0329) (-0.5712, -38.0711) (-0.6275, -38.1192) (-0.6774, -38.1737) (-0.7217, -38.2328) (-0.7732, -38.3167) (-0.8222, -38.4302) (-0.8777, -38.6192) (-0.9329, -38.8591) (-1.0168, -39.1423) (-1.1064, -39.4236) (-1.2364, -39.7953) (-1.4149, -40.2541) (-1.6524, -40.7949) (-1.9088, -41.3271) (-2.0953, -41.6739) (-2.1885, -41.8473) knots 0 0 0 0 0.059055 0.118109 0.177163 0.236216 0.265745 0.295273 0.3248 0.354329 0.36909 0.383846 0.391225 0.398597 0.405969 0.413352 0.420732 0.428104 0.435485 0.442861 0.472389 0.501917 0.509293 0.516674 0.524045 0.531426 0.538808 0.54618 0.553552 0.560931 0.575687 0.590449 0.619977 0.649505 0.679033 0.708561 0.767614 0.826668 0.885723 0.944777 0.944777 0.944777 0.944777
  spline S24 degree 3 poles (7.8664, -41.1595) (7.7504, -41.0004) (7.5184, -40.6823) (7.1919, -40.19) (6.883, -39.6865) (6.6436, -39.2563) (6.4643, -38.9058) (6.3372, -38.6393) (6.2155, -38.3701) (6.1281, -38.14) (6.0474, -37.9603) (5.9835, -37.8546) (5.921, -37.7784) (5.8691, -37.7259) (5.8123, -37.6787) (5.7499, -37.6387) (5.6818, -37.6096) (5.6108, -37.589) (5.5375, -37.5778) (5.3895, -37.5855) (5.1718, -37.6275) (4.9508, -37.6458) (4.8062, -37.6783) (4.7386, -37.7089) (4.6758, -37.7478) (4.6181, -37.7943) (4.5689, -37.8496) (4.5269, -37.9104) (4.4911, -37.975) (4.4514, -38.0651) (4.4184, -38.1842) (4.3891, -38.379) (4.3671, -38.6242) (4.3225, -38.9162) (4.272, -39.2071) (4.194, -39.593) (4.0796, -40.0719) (3.9179, -40.64) (3.7363, -41.2021) (3.5988, -41.5711) (3.5301, -41.7555) knots 0 0 0 0 0.059055 0.118109 0.177163 0.236216 0.265745 0.295273 0.3248 0.354329 0.36909 0.383846 0.391225 0.398597 0.405969 0.413352 0.420732 0.428104 0.435485 0.442861 0.472389 0.501917 0.509293 0.516674 0.524045 0.531426 0.538808 0.54618 0.553552 0.560931 0.575687 0.590449 0.619977 0.649505 0.679033 0.708561 0.767614 0.826668 0.885723 0.944777 0.944777 0.944777 0.944777
  spline S25 degree 3 poles (13.3976, -39.705) (13.2611, -39.5632) (12.988, -39.2796) (12.5975, -38.8363) (12.2229, -38.3797) (11.9272, -37.9861) (11.7018, -37.6632) (11.5396, -37.4165) (11.3823, -37.1664) (11.2645, -36.9503) (11.16, -36.7833) (11.0823, -36.6872) (11.01, -36.6203) (10.9514, -36.5753) (10.8887, -36.5363) (10.8215, -36.5052) (10.75, -36.4856) (10.6769, -36.4749) (10.6027, -36.4738) (10.4572, -36.5016) (10.2472, -36.5728) (10.0308, -36.6211) (9.892, -36.673) (9.8292, -36.7124) (9.7723, -36.7596) (9.7214, -36.8134) (9.6802, -36.8749) (9.6468, -36.9409) (9.6202, -37.0097) (9.5932, -37.1045) (9.5767, -37.227) (9.5742, -37.4239) (9.5858, -37.6698) (9.5814, -37.9651) (9.571, -38.2602) (9.5461, -38.6532) (9.498, -39.1431) (9.4152, -39.728) (9.3119, -40.3096) (9.2259, -40.6938) (9.1829, -40.8859) knots 0 0 0 0 0.059055 0.118109 0.177163 0.236216 0.265745 0.295273 0.3248 0.354329 0.36909 0.383846 0.391225 0.398597 0.405969 0.413352 0.420732 0.428104 0.435485 0.442861 0.472389 0.501917 0.509293 0.516674 0.524045 0.531426 0.538808 0.54618 0.553552 0.560931 0.575687 0.590449 0.619977 0.649505 0.679033 0.708561 0.767614 0.826668 0.885723 0.944777 0.944777 0.944777 0.944777
  spline S26 degree 3 poles (18.6793, -37.5109) (18.5248, -37.389) (18.2156, -37.1452) (17.7683, -36.7593) (17.335, -36.3579) (16.9885, -36.0082) (16.7213, -35.719) (16.527, -35.4967) (16.3371, -35.2703) (16.1909, -35.0723) (16.0647, -34.9211) (15.9747, -34.8365) (15.8939, -34.7801) (15.8298, -34.7434) (15.7623, -34.7133) (15.6915, -34.6916) (15.618, -34.682) (15.5442, -34.6813) (15.4705, -34.6904) (15.3301, -34.7377) (15.1318, -34.8369) (14.9239, -34.9141) (14.7935, -34.9844) (14.7366, -35.0321) (14.6867, -35.0865) (14.6436, -35.1468) (14.6111, -35.2134) (14.5871, -35.2832) (14.5701, -35.3551) (14.5562, -35.4526) (14.5566, -35.5762) (14.5809, -35.7716) (14.6259, -36.0136) (14.6617, -36.3069) (14.6916, -36.6006) (14.7205, -36.9933) (14.7395, -37.4852) (14.7372, -38.0759) (14.714, -38.6662) (14.6811, -39.0585) (14.6647, -39.2547) knots 0 0 0 0 0.059055 0.118109 0.177163 0.236216 0.265745 0.295273 0.3248 0.354329 0.36909 0.383846 0.391225 0.398597 0.405969 0.413352 0.420732 0.428104 0.435485 0.442861 0.472389 0.501917 0.509293 0.516674 0.524045 0.531426 0.538808 0.54618 0.553552 0.560931 0.575687 0.590449 0.619977 0.649505 0.679033 0.708561 0.767614 0.826668 0.885723 0.944777 0.944777 0.944777 0.944777
  spline S27 degree 3 poles (23.6131, -34.618) (23.4433, -34.5183) (23.1038, -34.3189) (22.6082, -33.9974) (22.1243, -33.6588) (21.7334, -33.3595) (21.4293, -33.1094) (21.2065, -32.9156) (20.9876, -32.7173) (20.8158, -32.541) (20.6702, -32.4084) (20.5694, -32.3368) (20.4818, -32.2919) (20.4132, -32.2643) (20.3423, -32.2437) (20.2692, -32.2319) (20.1951, -32.2323) (20.1218, -32.2417) (20.0501, -32.2607) (19.9175, -32.3267) (19.7345, -32.452) (19.539, -32.5568) (19.4194, -32.6442) (19.3696, -32.6991) (19.3275, -32.7599) (19.2931, -32.8255) (19.2699, -32.8958) (19.2556, -32.9683) (19.2486, -33.0418) (19.2481, -33.1403) (19.2653, -33.2627) (19.316, -33.453) (19.3935, -33.6866) (19.4689, -33.9723) (19.5385, -34.2592) (19.6207, -34.6443) (19.7065, -35.1291) (19.7846, -35.7145) (19.842, -36.3025) (19.8628, -36.6957) (19.8733, -36.8923) knots 0 0 0 0 0.059055 0.118109 0.177163 0.236216 0.265745 0.295273 0.3248 0.354329 0.36909 0.383846 0.391225 0.398597 0.405969 0.413352 0.420732 0.428104 0.435485 0.442861 0.472389 0.501917 0.509293 0.516674 0.524045 0.531426 0.538808 0.54618 0.553552 0.560931 0.575687 0.590449 0.619977 0.649505 0.679033 0.708561 0.767614 0.826668 0.885723 0.944777 0.944777 0.944777 0.944777
  spline S28 degree 3 poles (28.107, -31.0803) (27.9252, -31.0046) (27.5617, -30.8533) (27.027, -30.6023) (26.5014, -30.3327) (26.0734, -30.0894) (25.7381, -29.8831) (25.491, -29.7214) (25.2471, -29.5547) (25.0529, -29.4035) (24.8906, -29.2919) (24.781, -29.2347) (24.6881, -29.2022) (24.6164, -29.1842) (24.5433, -29.1734) (24.4693, -29.1717) (24.396, -29.1822) (24.3246, -29.2015) (24.2562, -29.23) (24.1338, -29.3135) (23.9695, -29.4625) (23.7902, -29.593) (23.6836, -29.6959) (23.6417, -29.7571) (23.6083, -29.823) (23.5831, -29.8926) (23.5698, -29.9655) (23.5655, -30.0393) (23.5685, -30.1131) (23.5814, -30.2107) (23.6151, -30.3296) (23.6913, -30.5112) (23.7999, -30.7321) (23.9135, -31.0048) (24.0215, -31.2796) (24.1553, -31.6499) (24.3064, -32.1185) (24.4634, -32.6879) (24.6004, -33.2625) (24.6746, -33.6492) (24.7117, -33.8426) knots 0 0 0 0 0.059055 0.118109 0.177163 0.236216 0.265745 0.295273 0.3248 0.354329 0.36909 0.383846 0.391225 0.398597 0.405969 0.413352 0.420732 0.428104 0.435485 0.442861 0.472389 0.501917 0.509293 0.516674 0.524045 0.531426 0.538808 0.54618 0.553552 0.560931 0.575687 0.590449 0.619977 0.649505 0.679033 0.708561 0.767614 0.826668 0.885723 0.944777 0.944777 0.944777 0.944777
  spline S29 degree 3 poles (32.0773, -26.9635) (31.8869, -26.9133) (31.5062, -26.8129) (30.9423, -26.6371) (30.3849, -26.4415) (29.9277, -26.2589) (29.5674, -26.1001) (29.3006, -25.9736) (29.0363, -25.8416) (28.8234, -25.7182) (28.6474, -25.6298) (28.531, -25.5881) (28.4345, -25.5685) (28.3611, -25.5605) (28.2872, -25.5597) (28.2136, -25.5681) (28.1424, -25.5885) (28.0744, -25.6173) (28.0104, -25.6549) (27.9005, -25.7542) (27.7581, -25.9243) (27.5982, -26.0779) (27.5066, -26.1943) (27.4734, -26.2607) (27.4493, -26.3306) (27.4338, -26.403) (27.4305, -26.477) (27.4363, -26.5506) (27.4493, -26.6233) (27.4755, -26.7183) (27.525, -26.8315) (27.6252, -27.0011) (27.7629, -27.2052) (27.9126, -27.4598) (28.057, -27.7174) (28.24, -28.066) (28.4534, -28.5096) (28.6866, -29.0523) (28.9005, -29.603) (29.0266, -29.976) (29.0897, -30.1625) knots 0 0 0 0 0.059055 0.118109 0.177163 0.236216 0.265745 0.295273 0.3248 0.354329 0.36909 0.383846 0.391225 0.398597 0.405969 0.413352 0.420732 0.428104 0.435485 0.442861 0.472389 0.501917 0.509293 0.516674 0.524045 0.531426 0.538808 0.54618 0.553552 0.560931 0.575687 0.590449 0.619977 0.649505 0.679033 0.708561 0.767614 0.826668 0.885723 0.944777 0.944777 0.944777 0.944777
  spline S30 degree 3 poles (35.4501, -22.3445) (35.2546, -22.3207) (34.8638, -22.2731) (34.2811, -22.1757) (33.7024, -22.0578) (33.2246, -21.9391) (32.846, -21.8309) (32.5645, -21.7419) (32.2847, -21.6472) (32.0569, -21.5539) (31.8705, -21.4903) (31.7495, -21.4648) (31.6512, -21.4585) (31.5774, -21.4606) (31.5041, -21.4699) (31.4323, -21.4882) (31.3646, -21.5181) (31.3011, -21.5559) (31.2429, -21.6019) (31.1475, -21.7153) (31.0296, -21.9031) (30.8921, -22.0771) (30.8172, -22.2049) (30.7934, -22.2752) (30.779, -22.3476) (30.7735, -22.4215) (30.7803, -22.4953) (30.7961, -22.5674) (30.8189, -22.6377) (30.8577, -22.7282) (30.9222, -22.8336) (31.0446, -22.988) (31.2087, -23.1714) (31.3917, -23.4033) (31.5699, -23.6388) (31.7986, -23.9593) (32.0705, -24.3697) (32.3753, -24.8756) (32.6622, -25.392) (32.838, -25.7443) (32.9259, -25.9205) knots 0 0 0 0 0.059055 0.118109 0.177163 0.236216 0.265745 0.295273 0.3248 0.354329 0.36909 0.383846 0.391225 0.398597 0.405969 0.413352 0.420732 0.428104 0.435485 0.442861 0.472389 0.501917 0.509293 0.516674 0.524045 0.531426 0.538808 0.54618 0.553552 0.560931 0.575687 0.590449 0.619977 0.649505 0.679033 0.708561 0.767614 0.826668 0.885723 0.944777 0.944777 0.944777 0.944777
  spline S31 degree 3 poles (38.1625, -17.3093) (37.9656, -17.3123) (37.5719, -17.3184) (36.9814, -17.3012) (36.392, -17.2633) (35.9025, -17.2107) (35.5127, -17.155) (35.2217, -17.1052) (34.9316, -17.0494) (34.6932, -16.9881) (34.4999, -16.9504) (34.3766, -16.9416) (34.2784, -16.9488) (34.2055, -16.9609) (34.1342, -16.9801) (34.0655, -17.008) (34.0025, -17.0468) (33.9447, -17.093) (33.8933, -17.1464) (33.8143, -17.2717) (33.723, -17.4739) (33.6105, -17.665) (33.5537, -17.8018) (33.5397, -17.8747) (33.5353, -17.9484) (33.5399, -18.0223) (33.5567, -18.0945) (33.5822, -18.1639) (33.6143, -18.2303) (33.6651, -18.3147) (33.7434, -18.4104) (33.8856, -18.5466) (34.0732, -18.706) (34.2861, -18.9108) (34.4946, -19.1198) (34.7649, -19.4062) (35.0901, -19.7758) (35.461, -20.2355) (35.8156, -20.708) (36.0377, -21.0331) (36.1487, -21.1956) knots 0 0 0 0 0.059055 0.118109 0.177163 0.236216 0.265745 0.295273 0.3248 0.354329 0.36909 0.383846 0.391225 0.398597 0.405969 0.413352 0.420732 0.428104 0.435485 0.442861 0.472389 0.501917 0.509293 0.516674 0.524045 0.531426 0.538808 0.54618 0.553552 0.560931 0.575687 0.590449 0.619977 0.649505 0.679033 0.708561 0.767614 0.826668 0.885723 0.944777 0.944777 0.944777 0.944777
  spline S32 degree 3 poles (40.164, -11.9516) (39.9694, -11.9814) (39.5802, -12.041) (38.9928, -12.1044) (38.4037, -12.1471) (37.9116, -12.1617) (37.5179, -12.1596) (37.2228, -12.1499) (36.9278, -12.1341) (36.6833, -12.1058) (36.4866, -12.0948) (36.3633, -12.1029) (36.267, -12.1234) (36.1964, -12.1453) (36.1284, -12.174) (36.0642, -12.211) (36.007, -12.2581) (35.9561, -12.3116) (35.9124, -12.3716) (35.8512, -12.5065) (35.7883, -12.7192) (35.7029, -12.9238) (35.6652, -13.0671) (35.6612, -13.1412) (35.6669, -13.2149) (35.6816, -13.2875) (35.7081, -13.3566) (35.7427, -13.4219) (35.7836, -13.4834) (35.8454, -13.5601) (35.936, -13.6442) (36.0954, -13.7598) (36.303, -13.8921) (36.5417, -14.0661) (36.7768, -14.2447) (37.0836, -14.4916) (37.4561, -14.8135) (37.8861, -15.2184) (38.3017, -15.6382) (38.566, -15.9301) (38.6982, -16.076) knots 0 0 0 0 0.059055 0.118109 0.177163 0.236216 0.265745 0.295273 0.3248 0.354329 0.36909 0.383846 0.391225 0.398597 0.405969 0.413352 0.420732 0.428104 0.435485 0.442861 0.472389 0.501917 0.509293 0.516674 0.524045 0.531426 0.538808 0.54618 0.553552 0.560931 0.575687 0.590449 0.619977 0.649505 0.679033 0.708561 0.767614 0.826668 0.885723 0.944777 0.944777 0.944777 0.944777
  spline S33 degree 3 poles (41.4173, -6.3713) (41.2286, -6.4273) (40.8511, -6.5394) (40.2779, -6.6821) (39.7, -6.8046) (39.2145, -6.8861) (38.8242, -6.9377) (38.5305, -6.9682) (38.2361, -6.9928) (37.99, -6.998) (37.7937, -7.0139) (37.6726, -7.0387) (37.58, -7.0721) (37.5131, -7.1034) (37.4496, -7.1412) (37.391, -7.1865) (37.3407, -7.2409) (37.2976, -7.3009) (37.2625, -7.3663) (37.2202, -7.5083) (37.1869, -7.7275) (37.1301, -7.9419) (37.1123, -8.089) (37.1185, -8.1629) (37.1342, -8.2351) (37.1586, -8.3051) (37.1942, -8.37) (37.2374, -8.4299) (37.2863, -8.4853) (37.358, -8.5528) (37.4592, -8.6238) (37.6329, -8.7166) (37.8565, -8.8195) (38.1167, -8.9593) (38.374, -9.1043) (38.7114, -9.3071) (39.1243, -9.5752) (39.6055, -9.9178) (40.0744, -10.2771) (40.376, -10.5303) (40.5267, -10.6568) knots 0 0 0 0 0.059055 0.118109 0.177163 0.236216 0.265745 0.295273 0.3248 0.354329 0.36909 0.383846 0.391225 0.398597 0.405969 0.413352 0.420732 0.428104 0.435485 0.442861 0.472389 0.501917 0.509293 0.516674 0.524045 0.531426 0.538808 0.54618 0.553552 0.560931 0.575687 0.590449 0.619977 0.649505 0.679033 0.708561 0.767614 0.826668 0.885723 0.944777 0.944777 0.944777 0.944777
  spline S34 degree 3 poles (41.8991, -0.6723) (41.7197, -0.7535) (41.361, -0.9159) (40.8126, -1.1354) (40.2568, -1.3354) (39.7869, -1.4823) (39.4072, -1.5865) (39.1204, -1.6567) (38.8322, -1.7212) (38.5891, -1.7598) (38.3968, -1.8023) (38.2802, -1.8434) (38.1929, -1.8891) (38.1309, -1.9292) (38.0731, -1.9753) (38.0213, -2.0282) (37.9789, -2.0889) (37.9444, -2.1542) (37.9185, -2.2238) (37.8959, -2.3702) (37.8927, -2.5919) (37.8657, -2.812) (37.8681, -2.9602) (37.8843, -3.0326) (37.9096, -3.102) (37.9433, -3.1679) (37.9875, -3.2274) (38.0385, -3.2809) (38.0944, -3.3291) (38.1746, -3.3863) (38.2845, -3.4428) (38.4693, -3.5111) (38.7048, -3.5825) (38.9817, -3.6856) (39.2562, -3.7942) (39.6182, -3.9492) (40.0637, -4.1586) (40.5871, -4.4325) (41.1005, -4.7246) (41.4338, -4.9343) (41.6004, -5.0392) knots 0 0 0 0 0.059055 0.118109 0.177163 0.236216 0.265745 0.295273 0.3248 0.354329 0.36909 0.383846 0.391225 0.398597 0.405969 0.413352 0.420732 0.428104 0.435485 0.442861 0.472389 0.501917 0.509293 0.516674 0.524045 0.531426 0.538808 0.54618 0.553552 0.560931 0.575687 0.590449 0.619977 0.649505 0.679033 0.708561 0.767614 0.826668 0.885723 0.944777 0.944777 0.944777 0.944777
  spline S35 degree 3 poles (41.6004, 5.0392) (41.4338, 4.9343) (41.1005, 4.7246) (40.5871, 4.4325) (40.0637, 4.1586) (39.6182, 3.9492) (39.2562, 3.7942) (38.9817, 3.6856) (38.7048, 3.5825) (38.4693, 3.5111) (38.2845, 3.4428) (38.1746, 3.3863) (38.0944, 3.3291) (38.0385, 3.2809) (37.9875, 3.2274) (37.9433, 3.1679) (37.9096, 3.102) (37.8843, 3.0326) (37.8681, 2.9602) (37.8657, 2.812) (37.8927, 2.5919) (37.8959, 2.3702) (37.9185, 2.2238) (37.9444, 2.1542) (37.9789, 2.0889) (38.0213, 2.0282) (38.0731, 1.9753) (38.1309, 1.9292) (38.1929, 1.8891) (38.2802, 1.8434) (38.3968, 1.8023) (38.5891, 1.7598) (38.8322, 1.7212) (39.1204, 1.6567) (39.4072, 1.5865) (39.7869, 1.4823) (40.2568, 1.3354) (40.8126, 1.1354) (41.361, 0.9159) (41.7197, 0.7535) (41.8991, 0.6723) knots 0 0 0 0 0.059055 0.118109 0.177163 0.236216 0.265745 0.295273 0.3248 0.354329 0.36909 0.383846 0.391225 0.398597 0.405969 0.413352 0.420732 0.428104 0.435485 0.442861 0.472389 0.501917 0.509293 0.516674 0.524045 0.531426 0.538808 0.54618 0.553552 0.560931 0.575687 0.590449 0.619977 0.649505 0.679033 0.708561 0.767614 0.826668 0.885723 0.944777 0.944777 0.944777 0.944777
  spline S36 degree 3 poles (40.5267, 10.6568) (40.376, 10.5303) (40.0744, 10.2771) (39.6055, 9.9178) (39.1243, 9.5752) (38.7114, 9.3071) (38.374, 9.1043) (38.1167, 8.9593) (37.8565, 8.8195) (37.6329, 8.7166) (37.4592, 8.6238) (37.358, 8.5528) (37.2863, 8.4853) (37.2374, 8.4299) (37.1942, 8.37) (37.1586, 8.3051) (37.1342, 8.2351) (37.1185, 8.1629) (37.1123, 8.089) (37.1301, 7.9419) (37.1869, 7.7275) (37.2202, 7.5083) (37.2625, 7.3663) (37.2976, 7.3009) (37.3407, 7.2409) (37.391, 7.1865) (37.4496, 7.1412) (37.5131, 7.1034) (37.58, 7.0721) (37.6726, 7.0387) (37.7937, 7.0139) (37.99, 6.998) (38.2361, 6.9928) (38.5305, 6.9682) (38.8242, 6.9377) (39.2145, 6.8861) (39.7, 6.8046) (40.2779, 6.6821) (40.8511, 6.5394) (41.2286, 6.4273) (41.4173, 6.3713) knots 0 0 0 0 0.059055 0.118109 0.177163 0.236216 0.265745 0.295273 0.3248 0.354329 0.36909 0.383846 0.391225 0.398597 0.405969 0.413352 0.420732 0.428104 0.435485 0.442861 0.472389 0.501917 0.509293 0.516674 0.524045 0.531426 0.538808 0.54618 0.553552 0.560931 0.575687 0.590449 0.619977 0.649505 0.679033 0.708561 0.767614 0.826668 0.885723 0.944777 0.944777 0.944777 0.944777
  spline S37 degree 3 poles (38.6982, 16.076) (38.566, 15.9301) (38.3017, 15.6382) (37.8861, 15.2184) (37.4561, 14.8135) (37.0836, 14.4916) (36.7768, 14.2447) (36.5417, 14.0661) (36.303, 13.8921) (36.0954, 13.7598) (35.936, 13.6442) (35.8454, 13.5601) (35.7836, 13.4834) (35.7427, 13.4219) (35.7081, 13.3566) (35.6816, 13.2875) (35.6669, 13.2149) (35.6612, 13.1412) (35.6652, 13.0671) (35.7029, 12.9238) (35.7883, 12.7192) (35.8512, 12.5065) (35.9124, 12.3716) (35.9561, 12.3116) (36.007, 12.2581) (36.0642, 12.211) (36.1284, 12.174) (36.1964, 12.1453) (36.267, 12.1234) (36.3633, 12.1029) (36.4866, 12.0948) (36.6833, 12.1058) (36.9278, 12.1341) (37.2228, 12.1499) (37.5179, 12.1596) (37.9116, 12.1617) (38.4037, 12.1471) (38.9928, 12.1044) (39.5802, 12.041) (39.9694, 11.9814) (40.164, 11.9516) knots 0 0 0 0 0.059055 0.118109 0.177163 0.236216 0.265745 0.295273 0.3248 0.354329 0.36909 0.383846 0.391225 0.398597 0.405969 0.413352 0.420732 0.428104 0.435485 0.442861 0.472389 0.501917 0.509293 0.516674 0.524045 0.531426 0.538808 0.54618 0.553552 0.560931 0.575687 0.590449 0.619977 0.649505 0.679033 0.708561 0.767614 0.826668 0.885723 0.944777 0.944777 0.944777 0.944777
  spline S38 degree 3 poles (36.1487, 21.1956) (36.0377, 21.0331) (35.8156, 20.708) (35.461, 20.2355) (35.0901, 19.7758) (34.7649, 19.4062) (34.4946, 19.1198) (34.2861, 18.9108) (34.0732, 18.706) (33.8856, 18.5466) (33.7434, 18.4104) (33.6651, 18.3147) (33.6143, 18.2303) (33.5822, 18.1639) (33.5567, 18.0945) (33.5399, 18.0223) (33.5353, 17.9484) (33.5397, 17.8747) (33.5537, 17.8018) (33.6105, 17.665) (33.723, 17.4739) (33.8143, 17.2717) (33.8933, 17.1464) (33.9447, 17.093) (34.0025, 17.0468) (34.0655, 17.008) (34.1342, 16.9801) (34.2055, 16.9609) (34.2784, 16.9488) (34.3766, 16.9416) (34.4999, 16.9504) (34.6932, 16.9881) (34.9316, 17.0494) (35.2217, 17.1052) (35.5127, 17.155) (35.9025, 17.2107) (36.392, 17.2633) (36.9814, 17.3012) (37.5719, 17.3184) (37.9656, 17.3123) (38.1625, 17.3093) knots 0 0 0 0 0.059055 0.118109 0.177163 0.236216 0.265745 0.295273 0.3248 0.354329 0.36909 0.383846 0.391225 0.398597 0.405969 0.413352 0.420732 0.428104 0.435485 0.442861 0.472389 0.501917 0.509293 0.516674 0.524045 0.531426 0.538808 0.54618 0.553552 0.560931 0.575687 0.590449 0.619977 0.649505 0.679033 0.708561 0.767614 0.826668 0.885723 0.944777 0.944777 0.944777 0.944777
  spline S39 degree 3 poles (32.9259, 25.9205) (32.838, 25.7443) (32.6622, 25.392) (32.3753, 24.8756) (32.0705, 24.3697) (31.7986, 23.9593) (31.5699, 23.6388) (31.3917, 23.4033) (31.2087, 23.1714) (31.0446, 22.988) (30.9222, 22.8336) (30.8577, 22.7282) (30.8189, 22.6377) (30.7961, 22.5674) (30.7803, 22.4953) (30.7735, 22.4215) (30.779, 22.3476) (30.7934, 22.2752) (30.8172, 22.2049) (30.8921, 22.0771) (31.0296, 21.9031) (31.1475, 21.7153) (31.2429, 21.6019) (31.3011, 21.5559) (31.3646, 21.5181) (31.4323, 21.4882) (31.5041, 21.4699) (31.5774, 21.4606) (31.6512, 21.4585) (31.7495, 21.4648) (31.8705, 21.4903) (32.0569, 21.5539) (32.2847, 21.6472) (32.5645, 21.7419) (32.846, 21.8309) (33.2246, 21.9391) (33.7024, 22.0578) (34.2811, 22.1757) (34.8638, 22.2731) (35.2546, 22.3207) (35.4501, 22.3445) knots 0 0 0 0 0.059055 0.118109 0.177163 0.236216 0.265745 0.295273 0.3248 0.354329 0.36909 0.383846 0.391225 0.398597 0.405969 0.413352 0.420732 0.428104 0.435485 0.442861 0.472389 0.501917 0.509293 0.516674 0.524045 0.531426 0.538808 0.54618 0.553552 0.560931 0.575687 0.590449 0.619977 0.649505 0.679033 0.708561 0.767614 0.826668 0.885723 0.944777 0.944777 0.944777 0.944777